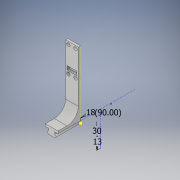
# Autodesk Inventor part: prox_base
Saved by Autodesk Inventor 2019.3 (Build 233278000, 278)
## iProperties
Created: 2019-04-13
Part Number: prox_base
Material: Generic
Document SubType Name: Modeling
Designer: peter
Density: 1 g/cm^3
Appearance: Default
Author: peter
Autodesk Inventor part; units mm, degrees
ref_plane "YZ Plane" through (0, 0, 0) normal (1, 0, 0) x (0, 1, 0)
ref_plane "XZ Plane" through (0, 0, 0) normal (0, 1, 0) x (-1, 0, 0)
ref_plane "XY Plane" through (0, 0, 0) normal (0, 0, 1) x (1, 0, 0)
sketch "Sketch1" plane through (0, 0, 0) normal (0, 0, 1) x (1, 0, 0)
  line L0 (-11.25, 59.5) -> (-8.75, 59.5) construction
  line L1 (-8.75, 59.5) -> (-8.75, 57) construction
  line L2 (-8.75, 57) -> (-11.25, 57) construction
  line L3 (-11.25, 57) -> (-11.25, 59.5) construction
  line L4 (0, 59.5) -> (-11.25, 59.5) construction
  circle A0 centre (-8.75, 57) radius 1.5
  line L5 (-8.75, 57) -> (-2.5, 57) construction
  line L6 (-2.5, 57) -> (-2.5, 34.5) construction
  line L7 (-2.5, 34.5) -> (-8.75, 34.5) construction
  line L8 (-8.75, 34.5) -> (-8.75, 57) construction
  circle A1 centre (-8.75, 34.5) radius 1.5
  circle A2 centre (-2.5, 34.5) radius 1.5
  circle A3 centre (-2.5, 57) radius 1.5
  line L9 (-11.25, 59.5) -> (0, 59.5)
  line L10 (0, 59.5) -> (0, 2)
  line L11 (0, 2) -> (-11.25, 2)
  line L12 (-11.25, 2) -> (-11.25, 59.5)
  line L13 (-9.95, 40.4) -> (0, 40.4) construction
  line L14 (-1.3, 40.4) -> (0, 40.4) construction
  line L15 (-9.95, 37) -> (0, 37) construction
  line L16 (-9.95, 40.4) -> (-1.3, 40.4)
  line L17 (-1.3, 40.4) -> (-1.3, 37)
  line L18 (-1.3, 37) -> (-9.95, 37)
  line L19 (-9.95, 37) -> (-9.95, 40.4)
  line L20 (0, 59.5) -> (-1.3, 59.5) construction
  line L21 (-1.3, 59.5) -> (-1.3, 40.4) construction
  line L22 (-1.3, 40.4) -> (0, 40.4) construction
  line L23 (0, 40.4) -> (0, 59.5) construction
  line L24 (0, 59.5) -> (-9.95, 59.5) construction
  line L25 (-9.95, 59.5) -> (-9.95, 37) construction
  line L26 (-9.95, 37) -> (0, 37) construction
  line L27 (0, 37) -> (0, 59.5) construction
  point P0 (0, 0)
  dimension "d0" = 2.5
  dimension "d1" = 2.5
  dimension "d2" = 3
  dimension "d3" = 6.25
  dimension "d4" = 22.5
  dimension "d5" = 3
  dimension "d6" = 3
  dimension "d7" = 3
  dimension "d8" = 11.25
  dimension "d9" = 57.5
  dimension "d10" = 9.95
  dimension "d11" = 1.3
  constraints: 56 end point, 12 parallel, 6 horizontal, 6 perpendicular, 4 centre point, 1 coincident, 1 point on line
  measures "d0" distance of L2.start L2.end
  measures "d1" distance of L1.start L2.start
  measures "d2" diameter of A0
  measures "d3" distance of L7.start L7.end
  measures "d4" distance of L6.start L7.start
  measures "d5" diameter of A1
  measures "d6" diameter of A2
  measures "d7" diameter of A3
  measures "d8" distance of L10.end L11.end
  measures "d9" distance of L9.end L10.end
  measures "d10" distance of L13.start L13.end
  measures "d11" distance of L14.start L14.end
extrude "Extrusion1" add sketch "Sketch1" along normal blind 2
sketch "Sketch2" plane through (0, 2, 0) normal (1, 0, 0) x (0, 0, -1)
  line L0 (0, 0) -> (0, 57.5) construction
  line L1 (0, 0) -> (18, 0) construction
  line L2 (18, 0) -> (18, -30) construction
  line L3 (18, 0) -> (48, 0) construction
  line L4 (18, -30) -> (18, -17) construction
  point P0 (0, -2)
  dimension "d14" = 18
  dimension "d15" = 30
  dimension "d16" = 90
  dimension "d17" = 13
  constraints: 8 end point, 2 horizontal, 1 perpendicular, 1 point on line, 1 vertical
  measures "d14" distance of L0.start L1.end
  measures "d15" distance of L1.end L2.end
  measures "d16" angle of L2 L3
  measures "d17" distance of L2.end L4.end
sketch "Sketch7" plane through (0, 0, 0) normal (0, 0, -1) x (-1, 0, 0)
  line L0 (1.4108, -1.2142) -> (2.825, -2.6284)
  line L1 (2.825, 0.2) -> (1.4108, -1.2142)
  line L2 (2.825, 0.2) -> (2.825, 2)
  line L3 (5.625, 0.2) -> (5.625, 2) construction
  line L4 (2.825, -2.6284) -> (5.625, -2.6284)
  line L5 (5.625, 2) -> (5.625, -3) construction
  line L6 (8.425, -2.6284) -> (5.625, -2.6284)
  line L7 (8.425, 0.2) -> (5.625, 0.2) construction
  line L8 (8.425, 2) -> (8.425, 0.2) construction
  line L9 (8.425, 2) -> (8.425, 0.2)
  line L10 (8.425, 0.2) -> (9.8392, -1.2142)
  line L11 (9.8392, -1.2142) -> (8.425, -2.6284)
  line L12 (8.425, 0.2) -> (10.425, 0.2) construction
  line L13 (9.95, 37) -> (1.3, 37) projected
  line L14 (1.3, 37) -> (1.3, 40.4) projected
  line L15 (1.3, 40.4) -> (9.95, 40.4) projected
  line L16 (9.95, 40.4) -> (9.95, 37) projected
  circle A0 centre (2.5, 57) radius 1.5 projected
  circle A1 centre (8.75, 57) radius 1.5 projected
  circle A2 centre (2.5, 34.5) radius 1.5 projected
  circle A3 centre (8.75, 34.5) radius 1.5 projected
  line L17 (11.25, 59.5) -> (0, 59.5) projected
  line L18 (0, 59.5) -> (0, 2) projected
  line L19 (0, 2) -> (11.25, 2) projected
  line L20 (11.25, 2) -> (11.25, 59.5) projected
  line L21 (11.25, 2) -> (0, 2) construction
  line L22 (5.625, 2) -> (5.625, 3.9478) construction
  line L23 (2.825, 2) -> (8.425, 2)
  line L24 (2.825, 2) -> (8.425, 2)
  line L25 (8.425, 2) -> (8.425, 0.2)
  line L26 (8.425, 0.2) -> (2.825, 0.2)
  line L27 (2.825, 0.2) -> (2.825, 2)
  line L28 (0, 2) -> (11.25, 2)
  line L29 (11.25, 2) -> (11.25, 4)
  line L30 (11.25, 4) -> (0, 4)
  line L31 (0, 4) -> (0, 2)
  dimension "d24" = 5
  dimension "d25" = 2.8
  dimension "d26" = 1.8
  dimension "d28" = 1.8
  dimension "d29" = 2
  dimension "d30" = 45
  dimension "d31" = 2
  dimension "d37" = 2
  constraints: 46 end point, 6 parallel, 5 perpendicular, 3 horizontal, 2 point on line, 2 symmetric about line, 2 vertical, 1 equal length, 1 midpoint
  measures "d24" distance of L3.end L5.end
  measures "d25" distance of L8.end L7.end
  measures "d26" distance of L8.start L8.end
  measures "d28" distance of L1.start L2.end
  measures "d29" distance of L8.end L10.end
  measures "d30" angle of L10 L12
  measures "d31" distance of L10.end L6.start
  measures "d37" distance of L29.end L28.end
extrude "Extrusion2" add sketch "Sketch7" against normal blind 20 contours L1 L26 L10 L11 L6 L4 L0 | L2 L19 L9 L26 | L19 L18 L30 L20
fillet "Fillet1" radius 10 1 edges at (-5.625, 4, 2)
body "Solid1"
